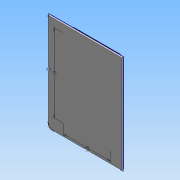
# Autodesk Inventor part: LCD12864
Saved by Autodesk Inventor 2016 (Build 200138000, 138)
## iProperties
Created: 2015-09-16
Part Number: LCD12864
Material: Generic
Document SubType Name: Modeling
Designer: Openlab
Density: 1 g/cm^3
Appearance: Default
Author: Openlab
Autodesk Inventor part; units mm, degrees
ref_plane "YZ Plane" through (0, 0, 0) normal (1, 0, 0) x (0, 1, 0)
ref_plane "XZ Plane" through (0, 0, 0) normal (0, 1, 0) x (-1, 0, 0)
ref_plane "XY Plane" through (0, 0, 0) normal (0, 0, 1) x (1, 0, 0)
sketch "Sketch1" plane through (0, 0, 0) normal (0, 1, 0) x (-1, 0, 0)
  line L0 (-35, 46.5) -> (35, 46.5)
  line L1 (35, 46.5) -> (35, -46.5)
  line L2 (35, -46.5) -> (-35, -46.5)
  line L3 (-35, -46.5) -> (-35, 46.5)
  line L4 (-35, 46.5) -> (35, -46.5) construction
  line L5 (35, 46.5) -> (-35, -46.5) construction
  line L6 (-22.5, 37.5) -> (22.5, 37.5)
  line L7 (22.5, 37.5) -> (22.5, -37.5)
  line L8 (22.5, -37.5) -> (-22.5, -37.5)
  line L9 (-22.5, -37.5) -> (-22.5, 37.5)
  line L10 (-22.5, 37.5) -> (22.5, -37.5) construction
  line L11 (22.5, 37.5) -> (-22.5, -37.5) construction
  point P0 (0, 0)
  dimension "d0" = 70
  dimension "d1" = 93
  dimension "d2" = 45
  dimension "d3" = 75
  constraints: 24 end point, 4 midpoint, 4 parallel, 2 horizontal, 2 perpendicular
  measures "d0" distance of L1.end L2.end
  measures "d1" distance of L0.end L1.end
  measures "d2" distance of L7.end L8.end
  measures "d3" distance of L6.end L7.end
extrude "Extrusion1" add sketch "Sketch1" against normal blind 1.6 contours L0 L1 L2 L3 | L6 L7 L8 L9
extrude "Extrusion2" add sketch "Sketch1" along normal blind 9.7 contours L6 L7 L8 L9
sketch "Sketch2" plane through (0, 9.7, 0) normal (0, 1, 0) x (1, 0, 0)
  line L0 (20, -35) -> (-20, -35)
  line L1 (-20, -35) -> (-20, 35)
  line L2 (-20, 35) -> (20, 35)
  line L3 (20, 35) -> (20, -35)
  line L4 (20, -35) -> (-20, 35) construction
  line L5 (-20, -35) -> (20, 35) construction
  point P0 (0, 0)
  dimension "d8" = 40
  dimension "d9" = 70
  constraints: 12 end point, 2 midpoint, 2 parallel, 1 horizontal, 1 perpendicular
  measures "d8" distance of L1.end L2.end
  measures "d9" distance of L0.end L1.end
extrude "Extrusion3" cut sketch "Sketch2" against normal blind 1
body "Solid1"
